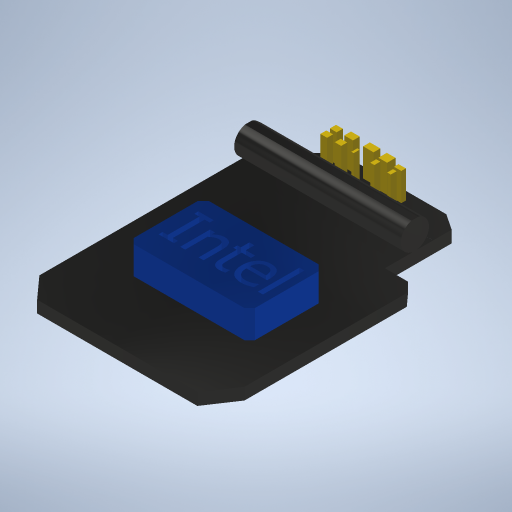
# Autodesk Inventor part: ARDUINO
Saved by Autodesk Inventor 2023 (Build 270158000, 158)
## iProperties
Created: 2022-10-20
Part Number: ARDUINO
Material: Generic
Document SubType Name: Modeling
Designer: Xiaba
Density: 1 g/cm^3
Appearance: Default
Author: Xiaba
Autodesk Inventor part; units mm, degrees
ref_plane "YZ Plane" through (0, 0, 0) normal (1, 0, 0) x (0, 1, 0)
ref_plane "XZ Plane" through (0, 0, 0) normal (0, 1, 0) x (-1, 0, 0)
ref_plane "XY Plane" through (0, 0, 0) normal (0, 0, 1) x (1, 0, 0)
sketch "Sketch1" plane through (0, 0, 0) normal (0, 1, 0) x (-1, 0, 0)
  line L0 (0, 0) -> (0.5, 0)
  line L1 (0.5, 0) -> (0.5, -0.7)
  line L2 (0.5, -0.7) -> (0, -0.7)
  line L3 (0, -0.7) -> (0, 0)
  dimension "d0" = 0.5
  dimension "d1" = 0.7
  constraints: 8 end point, 2 parallel, 1 horizontal, 1 perpendicular
  measures "d0" distance of L1.end L2.end
  measures "d1" distance of L0.end L1.end
extrude "Extrusion1" add sketch "Sketch1" along normal blind 0.1
sketch "Sketch2" plane through (0, 0.1, 0) normal (0, 1, 0) x (1, 0, 0)
  line L0 (0, 0.7) -> (-0.5, 0.7) projected
  line L1 (-0.5, 0.7) -> (-0.5, 0) projected
  line L2 (-0.5, 0) -> (0, 0) projected
  line L3 (0, 0) -> (0, 0.7) projected
  line L4 (-0.45, 0) -> (-0.5, 0.0556)
  line L5 (-0.5, 0.6262) -> (-0.426, 0.6262)
  line L6 (-0.426, 0.6262) -> (-0.426, 0.7)
  line L7 (-0.0473, 0) -> (0, 0.071)
  line L8 (0, 0.5052) -> (-0.0816, 0.5052)
  line L9 (-0.0816, 0.5052) -> (-0.0816, 0.7)
  line L10 (-0.426, 0.6631) -> (-0.385, 0.7)
  line L11 (-0.467, 0.6262) -> (-0.5, 0.5965)
  line L12 (-0.0816, 0.6733) -> (-0.1217, 0.7)
  line L13 (-0.0237, 0.5052) -> (0, 0.4789)
  constraints: 20 end point, 17 point on line, 5 perpendicular, 2 horizontal, 1 midpoint
extrude "Extrusion2" cut sketch "Sketch2" against normal blind 1 contours L3 L8 L9 L0 | L9 L12 L0 | L3 L13 L8 | L10 L6 L0 | L3 L2 L7 | L6 L5 L1 L0 | L2 L1 L4 | L5 L11 L1
sketch "Sketch3" plane through (-0.0816, 0.1, -0.5052) normal (1, 0, 0) x (0, 0, -1)
  circle A0 centre (0.0755, -0.0346) radius 0.0356
  line L0 (0.1111, 0.001) -> (0.0399, 0.001)
  line L1 (0.0399, 0.001) -> (0.0399, -0.0701)
  line L2 (0.0399, -0.0701) -> (0.1111, -0.0701)
  line L3 (0.1111, -0.0701) -> (0.1111, 0.001)
  line L4 (0.1111, 0.001) -> (0.0399, -0.0701) construction
  line L5 (0.0399, 0.001) -> (0.1111, -0.0701) construction
  line L6 (0.0399, 0.001) -> (0.1111, 0.001)
  line L7 (0.1111, 0.001) -> (0.1111, 0.0722)
  line L8 (0.1111, 0.0722) -> (0.0399, 0.0722)
  line L9 (0.0399, 0.0722) -> (0.0399, 0.001)
  point P0 (-0.5052, -0.1)
  point P1 (0.1111, -0.0346)
  point P2 (0.0755, -0.0701)
  point P3 (0.1111, 0.001)
  point P4 (0.0399, -0.0346)
  constraints: 20 end point, 4 parallel, 2 horizontal, 2 midpoint, 2 perpendicular, 1 centre point
extrude "Extrusion3" cut sketch "Sketch3" against normal blind 1 contours L3 L2 A0 | A0 L0 L3 | L0 L9 L8 L7 | A0 L1 L0 | L2 L1 A0
sketch "Sketch4" plane through (-0.0816, 0.1, -0.5722) normal (1, 0, 0) x (0, 0, -1)
  line L0 (0.0085, -0.0701) -> (-0.0271, -0.0701) projected
  line L1 (-0.0271, -0.0346) -> (-0.0271, 0) projected
  line L2 (-0.0271, 0) -> (-0.0371, 0)
  line L3 (-0.0371, 0) -> (-0.0371, -0.0701)
  line L4 (-0.0371, -0.0701) -> (-0.0271, -0.0701)
  line L5 (-0.0271, -0.0701) -> (-0.0271, 0)
  line L6 (0.054, 0) -> (0.0441, 0) projected
  line L7 (0.054, 0) -> (0.054, -0.1) projected
  line L8 (0.0441, 0) -> (0.054, 0)
  line L9 (0.054, 0) -> (0.054, -0.0701)
  line L10 (0.054, -0.0701) -> (0.0441, -0.0701)
  line L11 (0.0441, -0.0701) -> (0.0441, 0)
  point P0 (-0.5722, -0.1)
  dimension "d8" = 0.01
  dimension "d9" = 0.0099
  constraints: 16 end point, 4 parallel, 2 horizontal, 2 perpendicular, 1 point on line
  measures "d8" distance of L3.end L4.end
  measures "d9" distance of L9.end L10.end
extrude "Extrusion4" cut sketch "Sketch4" against normal blind 1
sketch "Sketch5" plane through (-0.0816, 0.1, -0.5722) normal (1, 0, 0) x (0, 0, -1)
  line L0 (0.001, -0.0626) -> (0.016, -0.0626)
  line L1 (0.016, -0.0626) -> (0.016, -0.0776)
  line L2 (0.016, -0.0776) -> (0.001, -0.0776)
  line L3 (0.001, -0.0776) -> (0.001, -0.0626)
  line L4 (0.001, -0.0626) -> (0.016, -0.0776) construction
  line L5 (0.016, -0.0626) -> (0.001, -0.0776) construction
  point P0 (-0.5722, -0.1)
  point P1 (0.0085, -0.0701)
  dimension "d12" = 0.015
  dimension "d13" = 0.015
  constraints: 12 end point, 2 midpoint, 2 parallel, 1 horizontal, 1 perpendicular
  measures "d12" distance of L1.end L2.end
  measures "d13" distance of L0.end L1.end
extrude "Extrusion5" add sketch "Sketch5" against normal blind 1
sketch "Sketch6" plane through (0, 0.1, 0) normal (0, 1, 0) x (1, 0, 0)
  line L0 (-0.3849, 0.6861) -> (-0.3679, 0.6861)
  line L1 (-0.3679, 0.6861) -> (-0.3679, 0.6705)
  line L2 (-0.3679, 0.6705) -> (-0.3849, 0.6705)
  line L3 (-0.3849, 0.6705) -> (-0.3849, 0.6861)
  line L4 (-0.3849, 0.6861) -> (-0.3679, 0.6705) construction
  line L5 (-0.3679, 0.6861) -> (-0.3849, 0.6705) construction
  line L6 (-0.3516, 0.6903) -> (-0.3296, 0.6903)
  line L7 (-0.3296, 0.6903) -> (-0.3296, 0.6733)
  line L8 (-0.3296, 0.6733) -> (-0.3516, 0.6733)
  line L9 (-0.3516, 0.6733) -> (-0.3516, 0.6903)
  line L10 (-0.3516, 0.6903) -> (-0.3296, 0.6733) construction
  line L11 (-0.3296, 0.6903) -> (-0.3516, 0.6733) construction
  line L12 (-0.3041, 0.6903) -> (-0.2779, 0.6903)
  line L13 (-0.2779, 0.6903) -> (-0.2779, 0.6733)
  line L14 (-0.2779, 0.6733) -> (-0.3041, 0.6733)
  line L15 (-0.3041, 0.6733) -> (-0.3041, 0.6903)
  line L16 (-0.3041, 0.6903) -> (-0.2779, 0.6733) construction
  line L17 (-0.2779, 0.6903) -> (-0.3041, 0.6733) construction
  line L18 (-0.2602, 0.6889) -> (-0.2382, 0.6889)
  line L19 (-0.2382, 0.6889) -> (-0.2382, 0.6677)
  line L20 (-0.2382, 0.6677) -> (-0.2602, 0.6677)
  line L21 (-0.2602, 0.6677) -> (-0.2602, 0.6889)
  line L22 (-0.2602, 0.6889) -> (-0.2382, 0.6677) construction
  line L23 (-0.2382, 0.6889) -> (-0.2602, 0.6677) construction
  line L24 (-0.2208, 0.679) -> (-0.2024, 0.679)
  line L25 (-0.2024, 0.679) -> (-0.2024, 0.6677)
  line L26 (-0.2024, 0.6677) -> (-0.2208, 0.6677)
  line L27 (-0.2208, 0.6677) -> (-0.2208, 0.679)
  line L28 (-0.2208, 0.679) -> (-0.2024, 0.6677) construction
  line L29 (-0.2024, 0.679) -> (-0.2208, 0.6677) construction
  line L30 (-0.3849, 0.6617) -> (-0.3679, 0.6617)
  line L31 (-0.3679, 0.6617) -> (-0.3679, 0.6466)
  line L32 (-0.3679, 0.6466) -> (-0.3849, 0.6466)
  line L33 (-0.3849, 0.6466) -> (-0.3849, 0.6617)
  line L34 (-0.3849, 0.6617) -> (-0.3679, 0.6466) construction
  line L35 (-0.3679, 0.6617) -> (-0.3849, 0.6466) construction
  line L36 (-0.3487, 0.6617) -> (-0.3325, 0.6617)
  line L37 (-0.3325, 0.6617) -> (-0.3325, 0.6466)
  line L38 (-0.3325, 0.6466) -> (-0.3487, 0.6466)
  line L39 (-0.3487, 0.6466) -> (-0.3487, 0.6617)
  line L40 (-0.3487, 0.6617) -> (-0.3325, 0.6466) construction
  line L41 (-0.3325, 0.6617) -> (-0.3487, 0.6466) construction
  line L42 (-0.3071, 0.6617) -> (-0.3011, 0.6617)
  line L43 (-0.3011, 0.6617) -> (-0.3011, 0.6466)
  line L44 (-0.3011, 0.6466) -> (-0.3071, 0.6466)
  line L45 (-0.3071, 0.6466) -> (-0.3071, 0.6617)
  line L46 (-0.3071, 0.6617) -> (-0.3011, 0.6466) construction
  line L47 (-0.3011, 0.6617) -> (-0.3071, 0.6466) construction
  line L48 (-0.2596, 0.6617) -> (-0.2492, 0.6617)
  line L49 (-0.2492, 0.6617) -> (-0.2492, 0.6466)
  line L50 (-0.2492, 0.6466) -> (-0.2596, 0.6466)
  line L51 (-0.2596, 0.6466) -> (-0.2596, 0.6617)
  line L52 (-0.2596, 0.6617) -> (-0.2492, 0.6466) construction
  line L53 (-0.2492, 0.6617) -> (-0.2596, 0.6466) construction
  line L54 (-0.2169, 0.6612) -> (-0.2079, 0.6612)
  line L55 (-0.2079, 0.6612) -> (-0.2079, 0.6466)
  line L56 (-0.2079, 0.6466) -> (-0.2169, 0.6466)
  line L57 (-0.2169, 0.6466) -> (-0.2169, 0.6612)
  line L58 (-0.2169, 0.6612) -> (-0.2079, 0.6466) construction
  line L59 (-0.2079, 0.6612) -> (-0.2169, 0.6466) construction
  line L60 (-0.3808, 0.3399) -> (-0.0994, 0.3399) construction
  line L61 (-0.0994, 0.3399) -> (-0.0994, 0.2333) construction
  line L62 (-0.0994, 0.2333) -> (-0.3808, 0.2333) construction
  line L63 (-0.3808, 0.2333) -> (-0.3808, 0.3399) construction
  line L64 (-0.3929, 0.3606) -> (-0.0881, 0.3606)
  line L65 (-0.0881, 0.3606) -> (-0.0881, 0.1722)
  line L66 (-0.0881, 0.1722) -> (-0.3929, 0.1722)
  line L67 (-0.3929, 0.1722) -> (-0.3929, 0.3606)
  line L68 (-0.0816, 0.5352) -> (-0.5, 0.5352) projected
  line L69 (-0.5, 0.5352) -> (-0.5, 0.0556) projected
  line L70 (-0.5, 0.0556) -> (-0.45, 0) projected
  line L71 (-0.45, 0) -> (-0.0473, 0) projected
  line L72 (-0.0473, 0) -> (0, 0.071) projected
  line L73 (0, 0.071) -> (0, 0.4789) projected
  line L74 (0, 0.4789) -> (-0.0237, 0.5052) projected
  line L75 (-0.0237, 0.5052) -> (-0.0816, 0.5052) projected
  line L76 (-0.0816, 0.5052) -> (-0.0816, 0.5352) projected
  line L77 (-0.426, 0.6262) -> (-0.0816, 0.6262) projected
  line L78 (-0.0816, 0.6262) -> (-0.0816, 0.6733) projected
  line L79 (-0.0816, 0.6733) -> (-0.1217, 0.7) projected
  line L80 (-0.1217, 0.7) -> (-0.385, 0.7) projected
  line L81 (-0.385, 0.7) -> (-0.426, 0.6631) projected
  line L82 (-0.426, 0.6631) -> (-0.426, 0.6262) projected
  point P0 (0, 0)
  point P1 (-0.3764, 0.6783)
  point P2 (-0.3406, 0.6818)
  point P3 (-0.291, 0.6818)
  point P4 (-0.2492, 0.6783)
  point P5 (-0.2116, 0.6733)
  point P6 (-0.3764, 0.6541)
  point P7 (-0.3406, 0.6541)
  point P8 (-0.3041, 0.6541)
  point P9 (-0.2544, 0.6541)
  point P10 (-0.2124, 0.6539)
  constraints: 128 end point, 22 parallel, 20 midpoint, 11 horizontal, 11 perpendicular, 7 point on line, 2 other
extrude "Extrusion6" cut sketch "Sketch6" against normal blind 0.07
sketch "Sketch7" plane through (0, 0.1, 0) normal (0, 1, 0) x (1, 0, 0)
  line L0 (-0.0881, 0.1722) -> (-0.0881, 0.3606) projected
  line L1 (-0.0881, 0.3606) -> (-0.3929, 0.3606) projected
  line L2 (-0.3929, 0.3606) -> (-0.3929, 0.1722) projected
  line L3 (-0.3929, 0.1722) -> (-0.0881, 0.1722) projected
  line L4 (-0.0881, 0.3606) -> (-0.3929, 0.3606) projected
  line L5 (-0.103, 0.3606) -> (-0.0881, 0.3459)
  line L6 (-0.0881, 0.1722) -> (-0.0881, 0.3606) projected
  line L7 (-0.0881, 0.1855) -> (-0.1012, 0.1722)
  line L8 (-0.3929, 0.1722) -> (-0.0881, 0.1722) projected
  line L9 (-0.3929, 0.3606) -> (-0.3929, 0.1722) projected
  line L10 (-0.3929, 0.1855) -> (-0.3794, 0.1722)
  line L11 (-0.3929, 0.3459) -> (-0.3784, 0.3606)
  line L12 (-0.3759, 0.3293) -> (-0.0981, 0.3293) construction
  line L13 (-0.0981, 0.3293) -> (-0.0981, 0.2231) construction
  line L14 (-0.0981, 0.2231) -> (-0.3759, 0.2231) construction
  line L15 (-0.3759, 0.2231) -> (-0.3759, 0.3293) construction
  line L16 (-0.3309, 0.2248) -> (-0.3696, 0.2248)
  line L17 (-0.3696, 0.2248) -> (-0.3696, 0.235)
  line L18 (-0.3696, 0.235) -> (-0.3569, 0.235)
  line L19 (-0.3569, 0.235) -> (-0.3569, 0.3146)
  line L20 (-0.3569, 0.3146) -> (-0.3696, 0.3146)
  line L21 (-0.3696, 0.3146) -> (-0.3696, 0.3248)
  line L22 (-0.3696, 0.3248) -> (-0.3309, 0.3248)
  line L23 (-0.3309, 0.3248) -> (-0.3309, 0.3146)
  line L24 (-0.3309, 0.3146) -> (-0.3436, 0.3146)
  line L25 (-0.3436, 0.3146) -> (-0.3436, 0.235)
  line L26 (-0.3436, 0.235) -> (-0.3309, 0.235)
  line L27 (-0.3309, 0.235) -> (-0.3309, 0.2248)
  line L28 (-0.2565, 0.2248) -> (-0.2691, 0.2248)
  line L29 (-0.2691, 0.2248) -> (-0.2691, 0.2676)
  spline S0 degree 2 poles (-0.2691, 0.2676) (-0.2691, 0.2728) (-0.2701, 0.2817) (-0.2716, 0.2844) knots 0 0 0 1 2 2 2
  spline S1 degree 2 poles (-0.2716, 0.2844) (-0.2731, 0.2872) (-0.2786, 0.29) (-0.2833, 0.29) knots 0 0 0 1 2 2 2
  spline S2 degree 2 poles (-0.2833, 0.29) (-0.288, 0.29) (-0.298, 0.2849) (-0.3028, 0.2809) knots 0 0 0 1 2 2 2
  line L30 (-0.3028, 0.2809) -> (-0.3028, 0.2248)
  line L31 (-0.3028, 0.2248) -> (-0.3154, 0.2248)
  line L32 (-0.3154, 0.2248) -> (-0.3154, 0.2998)
  line L33 (-0.3154, 0.2998) -> (-0.3028, 0.2998)
  line L34 (-0.3028, 0.2998) -> (-0.3028, 0.2915)
  spline S3 degree 2 poles (-0.3028, 0.2915) (-0.2971, 0.2966) (-0.2862, 0.302) (-0.28, 0.302) knots 0 0 0 1 2 2 2
  spline S4 degree 2 poles (-0.28, 0.302) (-0.269, 0.302) (-0.2565, 0.2874) (-0.2565, 0.2735) knots 0 0 0 1 2 2 2
  line L35 (-0.2565, 0.2735) -> (-0.2565, 0.2248)
  spline S5 degree 2 poles (-0.2161, 0.2233) (-0.2264, 0.2233) (-0.2379, 0.2351) (-0.2379, 0.2478) knots 0 0 0 1 2 2 2
  line L36 (-0.2379, 0.2478) -> (-0.2379, 0.2894)
  line L37 (-0.2379, 0.2894) -> (-0.2465, 0.2894)
  line L38 (-0.2465, 0.2894) -> (-0.2465, 0.2998)
  line L39 (-0.2465, 0.2998) -> (-0.2379, 0.2998)
  line L40 (-0.2379, 0.2998) -> (-0.2379, 0.3214)
  line L41 (-0.2379, 0.3214) -> (-0.2253, 0.3214)
  line L42 (-0.2253, 0.3214) -> (-0.2253, 0.2998)
  line L43 (-0.2253, 0.2998) -> (-0.202, 0.2998)
  line L44 (-0.202, 0.2998) -> (-0.202, 0.2894)
  line L45 (-0.202, 0.2894) -> (-0.2253, 0.2894)
  line L46 (-0.2253, 0.2894) -> (-0.2253, 0.2537)
  spline S6 degree 2 poles (-0.2253, 0.2537) (-0.2253, 0.248) (-0.2249, 0.2417) (-0.2235, 0.2391) knots 0 0 0 1 2 2 2
  spline S7 degree 2 poles (-0.2235, 0.2391) (-0.2224, 0.2367) (-0.2173, 0.2344) (-0.2129, 0.2344) knots 0 0 0 1 2 2 2
  spline S8 degree 2 poles (-0.2129, 0.2344) (-0.2098, 0.2344) (-0.2041, 0.2362) (-0.2028, 0.2368) knots 0 0 0 1 2 2 2
  line L47 (-0.2028, 0.2368) -> (-0.202, 0.2368)
  line L48 (-0.202, 0.2368) -> (-0.202, 0.2255)
  spline S9 degree 2 poles (-0.202, 0.2255) (-0.2056, 0.2245) (-0.2129, 0.2233) (-0.2161, 0.2233) knots 0 0 0 1 2 2 2
  spline S10 degree 2 poles (-0.1601, 0.2231) (-0.1781, 0.2231) (-0.1979, 0.2433) (-0.1979, 0.2619) knots 0 0 0 1 2 2 2
  spline S11 degree 2 poles (-0.1979, 0.2619) (-0.1979, 0.2802) (-0.1787, 0.302) (-0.1632, 0.302) knots 0 0 0 1 2 2 2
  spline S12 degree 2 poles (-0.1632, 0.302) (-0.1563, 0.302) (-0.1455, 0.2979) (-0.1415, 0.2936) knots 0 0 0 1 2 2 2
  spline S13 degree 2 poles (-0.1415, 0.2936) (-0.1375, 0.2893) (-0.1332, 0.2769) (-0.1332, 0.2679) knots 0 0 0 1 2 2 2
  line L49 (-0.1332, 0.2679) -> (-0.1332, 0.261)
  line L50 (-0.1332, 0.261) -> (-0.1851, 0.261)
  spline S14 degree 2 poles (-0.1851, 0.261) (-0.1851, 0.248) (-0.172, 0.2341) (-0.1603, 0.2341) knots 0 0 0 1 2 2 2
  spline S15 degree 2 poles (-0.1603, 0.2341) (-0.1562, 0.2341) (-0.1482, 0.236) (-0.1449, 0.2374) knots 0 0 0 1 2 2 2
  spline S16 degree 2 poles (-0.1449, 0.2374) (-0.1415, 0.2391) (-0.1368, 0.2419) (-0.1353, 0.2432) knots 0 0 0 1 2 2 2
  line L51 (-0.1353, 0.2432) -> (-0.1345, 0.2432)
  line L52 (-0.1345, 0.2432) -> (-0.1345, 0.2294)
  spline S17 degree 2 poles (-0.1345, 0.2294) (-0.1367, 0.2285) (-0.1434, 0.2259) (-0.146, 0.2252) knots 0 0 0 1 2 2 2
  spline S18 degree 2 poles (-0.146, 0.2252) (-0.1496, 0.2242) (-0.1556, 0.2231) (-0.1601, 0.2231) knots 0 0 0 1 2 2 2
  spline S19 degree 2 poles (-0.1455, 0.2707) (-0.1456, 0.2758) (-0.1478, 0.2832) (-0.1498, 0.2857) knots 0 0 0 1 2 2 2
  spline S20 degree 2 poles (-0.1498, 0.2857) (-0.152, 0.2886) (-0.1589, 0.2916) (-0.164, 0.2916) knots 0 0 0 1 2 2 2
  spline S21 degree 2 poles (-0.164, 0.2916) (-0.169, 0.2916) (-0.176, 0.2886) (-0.179, 0.2857) knots 0 0 0 1 2 2 2
  spline S22 degree 2 poles (-0.179, 0.2857) (-0.1818, 0.2827) (-0.1847, 0.2755) (-0.1851, 0.2707) knots 0 0 0 1 2 2 2
  line L53 (-0.1851, 0.2707) -> (-0.1455, 0.2707)
  line L54 (-0.1075, 0.2248) -> (-0.1201, 0.2248)
  line L55 (-0.1201, 0.2248) -> (-0.1201, 0.3293)
  line L56 (-0.1201, 0.3293) -> (-0.1075, 0.3293)
  line L57 (-0.1075, 0.3293) -> (-0.1075, 0.2248)
  point P0 (0, 0)
  constraints: 8 end point, 8 point on line, 3 perpendicular, 2 other
extrude "Extrusion7" cut sketch "Sketch7" against normal blind 0.07 contours L3 L7 L0 | L5 L1 L0 | L3 L2 L10 | L11 L2 L1 | L16 L17 L18 L19 L20 L21 L22 L23 L24 L25 L26 L27 | L28 L29 S0 S1 S2 L30 L31 L32 L33 L34 S3 S4 L35 | S5 L36 L37 L38 L39 L40 L41 L42 L43 L44 L45 L46 S6 S7 S8 L48 S9 | S10 S11 S12 S13 L49 L50 S14 S15 S16 L52 S17 S18 | L54 L55 L56 L57
sketch "Sketch8" plane through (-1.0816, 0.0374, -0.5882) normal (0, 1, 0) x (1, 0, 0)
  line L0 (0.5816, 0) -> (0.5816, -0.015) projected
  line L1 (0.5816, 0) -> (0, 0) projected
  line L2 (0, -0.015) -> (0, 0) projected
  line L3 (0.5816, -0.015) -> (0, -0.015) projected
  line L4 (0.5816, 0.0083) -> (0.5816, -0.5326) projected
  line L5 (-0.0114, 0.0274) -> (0.5816, 0.0274)
  line L6 (0.5816, 0.0274) -> (0.5816, -0.1715)
  line L7 (0.5816, -0.1715) -> (-0.0114, -0.1715)
  line L8 (-0.0114, -0.1715) -> (-0.0114, 0.0274)
  point P0 (1.0816, -0.5882)
  constraints: 8 end point, 2 parallel, 1 horizontal, 1 perpendicular, 1 point on line
extrude "Extrusion8" cut sketch "Sketch8" against normal blind 0.07
body "Solid1"
